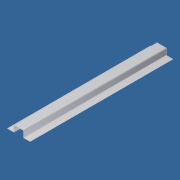
# Autodesk Inventor part: GE-12058
Saved by Autodesk Inventor 2012 (Build 160160000, 160)
## iProperties
Created: 2011-06-20
Part Number: GE-12058
Document SubType Name: Modeling
Designer: dfoster
Density: 1 g/cm^3
Description: Center Field Channel
Material: Default
Title: Center Field Channel
Author: dfoster
Autodesk Inventor part; units mm, degrees
ref_plane "YZ Plane" through (0, 0, 0) normal (1, 0, 0) x (0, 1, 0)
ref_plane "XZ Plane" through (0, 0, 0) normal (0, 1, 0) x (-1, 0, 0)
ref_plane "XY Plane" through (0, 0, 0) normal (0, 0, 1) x (1, 0, 0)
sketch "Sketch1" plane through (0, 0, 0) normal (0, 0, 1) x (1, 0, 0)
  line L0 (0, 6.223) -> (0, 95.25)
  line L1 (6.35, 101.6) -> (146.05, 101.6)
  line L2 (152.4, 95.25) -> (152.4, 6.223)
  arc A0 (6.35, 101.6) -> (0, 95.25) centre (6.35, 95.25) ccw
  arc A1 (152.4, 95.25) -> (146.05, 101.6) centre (146.05, 95.25) ccw
  line L3 (149.3622, 3.175) -> (149.3622, 95.25)
  arc A2 (149.3622, 95.25) -> (146.05, 98.5622) centre (146.05, 95.25) ccw
  line L4 (146.05, 98.5622) -> (6.35, 98.5622)
  arc A3 (6.35, 98.5622) -> (3.0378, 95.25) centre (6.35, 95.25) ccw
  line L5 (3.0378, 95.25) -> (3.0378, 3.175)
  line L6 (-0.1372, 0) -> (-101.6, 0)
  line L7 (-101.6, 0) -> (-101.6, 3.048)
  line L8 (-101.6, 3.048) -> (-3.175, 3.048)
  arc A4 (-3.175, 3.048) -> (0, 6.223) centre (-3.175, 6.223) ccw
  arc A5 (-0.1372, 0) -> (3.0378, 3.175) centre (-0.1372, 3.175) ccw
  line L9 (152.5372, 0) -> (254, 0)
  line L10 (254, 0) -> (254, 3.048)
  line L11 (254, 3.048) -> (155.575, 3.048)
  arc A6 (152.4, 6.223) -> (155.575, 3.048) centre (155.575, 6.223) ccw
  arc A7 (149.3622, 3.175) -> (152.5372, 0) centre (152.5372, 3.175) ccw
  point P0 (0, 0)
  point P1 (152.4, 3.048)
  point P2 (149.3622, 0)
  point P3 (3.0378, 0)
  dimension "d0" = 6.35
  dimension "d1" = 3.0378
  dimension "d2" = 152.4
  dimension "d6" = 3.048
  dimension "d7" = 101.6
  dimension "d8" = 3.175
  dimension "d9" = 101.6
  dimension "d10" = 3.048
  dimension "d11" = 3.175
  dimension "d12" = 101.6
  dimension "d13" = 101.6
  constraints: 24 end point, 16 point on circle, 12 tangent, 8 centre point, 6 point on line, 5 parallel, 5 perpendicular, 3 equal radius, 1 vertical, 2 other
  measures "d0" radius of A0
  measures "d1" distance between parallel lines of L4 L1
  measures "d2" distance between parallel lines of L2 L0
  measures "d6" distance between parallel lines of L6 L8
  measures "d7" distance from line of L0 L7.end
  measures "d8" radius of A4
  measures "d9" distance between parallel lines of L10 L2
  measures "d10" distance between parallel lines of L9 L11
  measures "d11" radius of A6
  measures "d12" distance between parallel lines of L9 L1
  measures "d13" distance between parallel lines of L6 L1
extrude "Extrusion1" add sketch "Sketch1" along normal blind 2235.2
body "Solid1"
